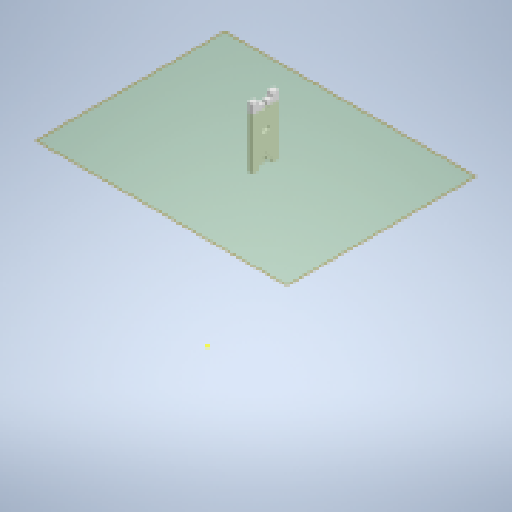
# Autodesk Inventor part: стенка 2
Saved by Autodesk Inventor 2024.2 (Build 282272000, 272)
## iProperties
Created: 2025-12-09
Part Number: стенка 2
Material: Типовые
Document SubType Name: Modeling
Designer: katya_notebook
Density: 1 g/cm^3
Appearance: По умолчанию
Author: katya_notebook
Autodesk Inventor part; units mm, degrees
ref_plane "YZ Plane" through (0, 0, 0) normal (1, 0, 0) x (0, 1, 0)
ref_plane "XZ Plane" through (0, 0, 0) normal (0, 1, 0) x (-1, 0, 0)
ref_plane "XY Plane" through (0, 0, 0) normal (0, 0, 1) x (1, 0, 0)
ref_plane "РабПлоскость1" through (-329.2239, 210.3045, -11.0538) normal (0, -1, 0) x (1, 0, 0)
sketch "Эскиз1" plane through (-329.2239, 210.3045, -11.0538) normal (0, -1, 0) x (1, 0, 0)
  line L0 (-46.5606, -73) -> (-52.5606, -73)
  line L1 (-52.5606, -73) -> (-52.5606, -43)
  line L2 (-52.5606, -43) -> (-46.5606, -43)
  line L3 (-46.5606, -43) -> (-46.5606, -73)
  line L4 (-23.55, -78) -> (-51.55, -78) projected
  point P0 (329.2239, 11.0538)
  dimension "d0" = 6
  dimension "d1" = 30
  dimension "d2" = 5
  constraints: 8 end point, 2 parallel, 1 horizontal, 1 perpendicular
  measures "d0" distance of L1.end L2.end
  measures "d1" distance of L0.end L1.end
  measures "d2" distance from line of L4 L0.start
ref_plane "РабПлоскость2" through (-464.2239, 154.5996, -124.0538) normal (0, 1, 0) x (0, 0, 1)
extrude "Выдавливание1" add sketch "Эскиз1" along normal blind 55.705 and the other way blind 5.645
sketch "Эскиз2" plane through (-375.7846, 215.9495, -54.0538) normal (1, 0, 0) x (0, 0, -1)
  line L0 (30, 0) -> (30, -61.35) projected
  line L1 (30, -30.675) -> (0, -30.675)
  line L2 (0, 0) -> (0, -61.35) projected
  line L3 (30, 0) -> (23, 0)
  line L4 (23, 0) -> (23, 5)
  line L5 (23, 5) -> (30, 5)
  line L6 (30, 5) -> (30, 0)
  line L7 (0, 0) -> (7, 0)
  line L8 (7, 0) -> (7, 5)
  line L9 (7, 5) -> (0, 5)
  line L10 (0, 5) -> (0, 0)
  line L11 (18.25, -4.5) -> (11.75, -4.5)
  line L12 (11.75, -4.5) -> (11.75, -7)
  line L13 (11.75, -7) -> (18.25, -7)
  line L14 (18.25, -7) -> (18.25, -4.5)
  line L15 (13.25, -9.1998) -> (16.75, -9.1998)
  line L16 (16.75, -9.1998) -> (16.75, 2.1998)
  line L17 (16.75, 2.1998) -> (13.25, 2.1998)
  line L18 (13.25, 2.1998) -> (13.25, -9.1998)
  line L19 (13.25, -9.1998) -> (16.75, 2.1998) construction
  line L20 (16.75, -9.1998) -> (13.25, 2.1998) construction
  line L21 (30, -61.35) -> (23, -61.35)
  line L22 (23, -61.35) -> (23, -66.35)
  line L23 (23, -66.35) -> (30, -66.35)
  line L24 (30, -66.35) -> (30, -61.35)
  line L25 (0, -61.35) -> (7, -61.35)
  line L26 (7, -61.35) -> (7, -66.35)
  line L27 (7, -66.35) -> (0, -66.35)
  line L28 (0, -66.35) -> (0, -61.35)
  line L29 (18.25, -54.35) -> (18.25, -56.85)
  line L30 (16.75, -63.5498) -> (13.25, -63.5498)
  line L31 (16.75, -52.1502) -> (16.75, -63.5498)
  line L32 (13.25, -52.1502) -> (16.75, -52.1502)
  line L33 (13.25, -52.1502) -> (16.75, -63.5498) construction
  line L34 (13.25, -63.5498) -> (13.25, -52.1502)
  line L35 (16.75, -52.1502) -> (13.25, -63.5498) construction
  line L36 (18.25, -56.85) -> (11.75, -56.85)
  line L37 (11.75, -56.85) -> (11.75, -54.35)
  line L38 (11.75, -54.35) -> (18.25, -54.35)
  point P0 (-54.0538, -215.9495)
  point P1 (0, -55.705)
  point P2 (30, -55.705)
  point P3 (15, -3.5)
  point P4 (16.75, -7)
  point P5 (16.75, -4.5)
  point P6 (13.25, -4.5)
  point P7 (13.25, -7)
  point P8 (15, -57.85)
  point P9 (16.75, -56.85)
  point P10 (16.75, -54.35)
  point P11 (13.25, -54.35)
  point P12 (13.25, -56.85)
  dimension "d23" = 5
  dimension "d24" = 7
  dimension "d25" = 7
  constraints: 74 end point, 15 symmetric about line, 4 parallel, 2 horizontal, 2 midpoint, 2 perpendicular
  measures "d23" distance of L5.end L0.start
  measures "d24" distance of L4.end L5.end
  measures "d25" distance of L8.end L9.end
extrude "Выдавливание2" add sketch "Эскиз2" against normal blind 6 contours L3 L4 L5 L6 | L10 L9 L8 L7 | L24 L23 L22 L21 | L25 L26 L27 L28
extrude "Выдавливание3" cut sketch "Эскиз2" against normal blind 6 contours L14 L13 L16 L11 | L16 L13 L18 L11 | L11 L18 L17 L16 | L18 L13 L12 L11 | L16 L15 L18 L13 | L29 L36 L31 L38 | L38 L34 L32 L31 | L31 L36 L34 L38 | L31 L30 L34 L36 | L34 L36 L37 L38
sketch "Эскиз5" plane through (-381.7846, 149.5996, -54.0538) normal (-1, 0, 0) x (0, 0, 1)
  line L0 (-20.1539, 35.705) -> (-10.1539, 35.705)
  line L1 (-10.1539, 39.705) -> (-20.1539, 39.705)
  line L2 (-10.1539, 35.705) -> (-10.1539, 39.705)
  line L3 (-20.1539, 39.705) -> (-20.1539, 35.705)
  point P0 (54.0538, -149.5996)
  constraints: 8 end point, 8 other
extrude "Выдавливание4" cut sketch "Эскиз5" against normal blind 10
